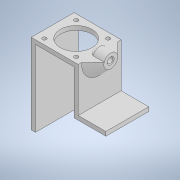
# Autodesk Inventor part: Motor Mount
Saved by Autodesk Inventor 2022 (Build 260153000, 153)
## iProperties
Created: 2022-04-23
Part Number: Motor Mount
Material: Generic
Document SubType Name: Modeling
Designer: Nick
Density: 1 g/cm^3
Appearance: Default
Author: Nick
Autodesk Inventor part; units mm, degrees
ref_plane "YZ Plane" through (0, 0, 0) normal (1, 0, 0) x (0, 1, 0)
ref_plane "XZ Plane" through (0, 0, 0) normal (0, 1, 0) x (-1, 0, 0)
ref_plane "XY Plane" through (0, 0, 0) normal (0, 0, 1) x (1, 0, 0)
sketch "Sketch1" plane through (0, 0, 0) normal (0, 0, 1) x (1, 0, 0)
  line L0 (0, 0) -> (0, 58.05)
  line L1 (0, 58.05) -> (34, 58.05)
  line L2 (34, 58.05) -> (34, 26.05)
  line L3 (34, 26.05) -> (54, 26.05)
  line L4 (54, 26.05) -> (54, 23.05)
  line L5 (54, 23.05) -> (31, 23.05)
  line L6 (31, 23.05) -> (31, 55.05)
  line L7 (31, 55.05) -> (3, 55.05)
  line L8 (3, 55.05) -> (3, 0)
  line L9 (3, 0) -> (0, 0)
  dimension "d0" = 3
  dimension "d1" = 3
  dimension "d2" = 3
  dimension "d3" = 28
  dimension "d4" = 55.05
  dimension "d5" = 3
  dimension "d6" = 32
  dimension "d7" = 20
  constraints: 20 end point, 6 perpendicular, 3 vertical, 1 parallel
  measures "d0" distance of L8.end L0.start
  measures "d1" distance between parallel lines of L1 L7
  measures "d2" distance between parallel lines of L2 L6
  measures "d3" distance of L6.end L7.end
  measures "d4" distance of L7.end L8.end
  measures "d5" distance of L3.end L4.end
  measures "d6" distance of L5.end L6.end
  measures "d7" distance of L2.end L3.end
extrude "Extrusion1" add sketch "Sketch1" along normal blind 31
sketch "Sketch2" plane through (0, 58.05, 0) normal (0, 1, 0) x (1, 0, 0)
  line L0 (5.5, -27) -> (28.5, -27) construction
  line L1 (28.5, -27) -> (28.5, -4) construction
  line L2 (28.5, -4) -> (5.5, -4) construction
  line L3 (5.5, -4) -> (5.5, -27) construction
  line L4 (0, 0) -> (0, -31) construction
  line L5 (34, 0) -> (0, 0) construction
  point P0 (17, -15.5)
  point P1 (5.5, -15.5)
  point P2 (0, -15.5)
  point P3 (17, -4)
  point P4 (17, 0)
  dimension "d10" = 23
  constraints: 8 end point, 4 midpoint, 2 coincident, 2 horizontal alignment, 2 parallel, 2 perpendicular, 2 vertical alignment, 1 horizontal
  measures "d10" distance of L2.end L0.start
hole "Hole1" at (5.5, 58.05, 27) at (5.5, 58.05, 4) at (28.5, 58.05, 4) at (28.5, 58.05, 27) direction (0, -1, 0) diameter 2.9 end through all clearance for "Socket Head Cap Screw" size "M2.5" standard "Ansi Metric M Profile"
hole "Hole2" at (17, 58.05, 15.5) direction (0, -1, 0) diameter 23 end through all
sketch "Sketch3" plane through (34, 26.05, 0) normal (1, 0, 0) x (0, 0, -1)
  circle A0 centre (-15.5, 30.5) radius 2
  line L0 (0, -3) -> (-31, -3) projected
  circle A1 centre (-15.5, 30.5) radius 5
  point P0 (0, -26.05)
  point P1 (-15.5, -3)
  dimension "d25" = 33.5
  dimension "d26" = 4
  dimension "d27" = 3
  constraints: 2 centre point, 1 midpoint, 1 vertical alignment
  measures "d25" distance from line of A0.centre L0
  measures "d26" diameter of A0
  measures "d27" radial gap between concentric circles of A0 A1
extrude "Extrusion2" add sketch "Sketch3" along normal blind 8
sketch "Sketch4" plane through (34, 26.05, 0) normal (-1, 0, 0) x (0, 0, 1)
  line L0 (16.8229, 32) -> (20.2697, 32) projected
  arc A0 (20.2697, 32) -> (10.7303, 32) centre (15.5, 30.5) ccw projected
  line L1 (10.7303, 32) -> (14.1771, 32) projected
  arc A1 (16.8229, 32) -> (14.1771, 32) centre (15.5, 30.5) ccw projected
  point P0 (0, -26.05)
revolve "Revolution1" add sketch "Sketch4" angle 90 about axis through (34, 58.05, 10.7303) along (0, 0, 1)
chamfer "Chamfer1" distance 8 angle 45 2 edges at (34, 57.3088, 10.5579) (34, 51.6079, 16.2588)
chamfer "Chamfer2" distance 0.5 angle 45 1 edges at (42, 56.55, 17.5)
body "Solid1"
